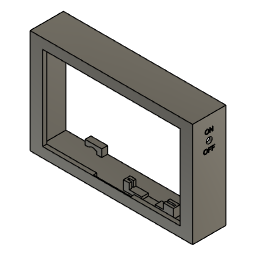
display (Autodesk Fusion 360 design; units mm, degrees)
Autodesk Fusion 360 part; units mm, degrees
note: some values were not read from the file. Set by a fixed rule: which face or edge a step refers to.
sketch "Outer" plane through (0, 0, 0) normal (0, 1, 0) x (1, 0, 0)
  line L0 (0, -125) -> (195, -125)
  line L1 (195, -125) -> (195, 0)
  line L2 (195, 0) -> (0, 0)
  line L3 (0, 0) -> (0, -125)
  line L4 (0, -62.5) -> (195, -62.5) construction
  line L5 (97.5, -125) -> (97.5, 0) construction
  dimension "d1" = 125
  dimension "d42" = 195
  constraint horizontal L0
  constraint vertical L1
  constraint horizontal L2
  constraint vertical L3
  constraint coincident L2.end L3.start
  constraint midpoint L3 L4.start
  constraint midpoint L1 L4.end
  constraint midpoint L0 L5.start
  constraint midpoint L2 L5.end
  measures "d1" distance of L0.start L2.end
  measures "d42" distance of L0.start L0.end
extrude "Extrude2" add sketch "Outer" along normal blind 40
shell "Shell1" thickness 3 removed faces 1 at (65, 40, 83.3333)
sketch "Screen Hole" plane through (0, 0, 0) normal (0, 1, 0) x (1, 0, 0)
  line L0 (15, -113) -> (180, -113)
  line L1 (180, -113) -> (180, -12)
  line L2 (180, -12) -> (15, -12)
  line L3 (15, -12) -> (15, -113)
  line L4 (0, -62.5) -> (195, -62.5)
  line L5 (0, 0) -> (0, -125)
  line L6 (3, -3) -> (3, -122)
  line L7 (192, -122) -> (192, -3)
  line L8 (97.5, -125) -> (97.5, 0)
  dimension "d10" = 165
  dimension "d11" = 101
  constraint horizontal L0
  constraint vertical L1
  constraint horizontal L2
  constraint vertical L3
  constraint symmetric L0 L2 L4
  constraint symmetric L1 L3 L8
  measures "d10" distance of L0.start L0.end
  measures "d11" distance of L0.start L2.end
extrude "Extrude3" cut sketch "Screen Hole" along normal blind 10
move_face "OffsetFaces1" offset 2 1 faces at (7, 3, 45.6667)
sketch "Cable Wedge" plane through (0, 5, 0) normal (0, 1, 0) x (-1, 0, 0)
  line L0 (-15, 12) -> (-180, 12)
  line L1 (-180, 12) -> (-180, 113)
  line L2 (-180, 113) -> (-15, 113)
  line L3 (-15, 113) -> (-15, 12)
  line L4 (-3, 3) -> (-3, 122)
  line L5 (-3, 122) -> (-192, 122)
  line L6 (-192, 122) -> (-192, 3)
  line L7 (-192, 3) -> (-3, 3)
  line L8 (-120, 12) -> (-75, 12)
  line L9 (-75, 12) -> (-75, 8)
  line L10 (-75, 8) -> (-120, 8)
  line L11 (-120, 8) -> (-120, 12)
  line L12 (-180, 113) -> (-180, 12)
  dimension "d43" = 60
  dimension "d44" = 45
  dimension "d45" = 4
  constraint horizontal L8
  constraint vertical L9
  constraint horizontal L10
  constraint vertical L11
  constraint coincident L0 L8.start
  measures "d43" distance of L11 L12
  measures "d44" distance of L9 L11
  measures "d45" distance of L8.start L10.end
extrude "Extrude6" cut sketch "Cable Wedge" against normal blind 4 contours L0 L8 L9 L10 L11
sketch "Screw Holes" plane through (0, 5, 0) normal (0, 1, 0) x (-1, 0, 0)
  line L0 (-120, 12) -> (-180, 12)
  line L1 (-180, 12) -> (-180, 113)
  line L2 (-180, 113) -> (-15, 113)
  line L3 (-15, 113) -> (-15, 12)
  line L4 (-3, 3) -> (-3, 122)
  line L5 (-3, 122) -> (-192, 122)
  line L6 (-192, 122) -> (-192, 3)
  line L7 (-192, 3) -> (-3, 3)
  circle A0 centre (-18.937, 8.19) radius 1.219
  circle A1 centre (-176.063, 8.19) radius 1.219
  circle A2 centre (-176.063, 116.81) radius 1.219
  circle A3 centre (-18.937, 116.81) radius 1.219
  line L8 (-120, 8) -> (-120, 12)
  line L9 (-15, 12) -> (-75, 12)
  line L10 (-75, 12) -> (-75, 8)
  line L11 (-75, 8) -> (-120, 8)
  dimension "d16" = 2.438
  dimension "d24" = 3.81
  dimension "d26" = 2.438
  dimension "d28" = 3.937
  dimension "d29" = 3.937
  dimension "d30" = 3.81
  dimension "d31" = 2.438
  dimension "d32" = 3.81
  dimension "d33" = 3.937
  dimension "d34" = 2.438
  dimension "d35" = 3.81
  dimension "d36" = 3.937
  measures "d16" diameter of A0
  measures "d24" distance of L0 A0.centre
  measures "d26" diameter of A1
  measures "d28" distance of L3 A0.centre
  measures "d29" distance of L1 A1.centre
  measures "d30" distance of L0 A1.centre
  measures "d31" diameter of A2
  measures "d32" distance of L2 A2.centre
  measures "d33" distance of L1 A2.centre
  measures "d34" diameter of A3
  measures "d35" distance of L2 A3.centre
  measures "d36" distance of L3 A3.centre
extrude "Extrude5" cut sketch "Screw Holes" against normal blind 4 contours A0 | A1 | A2 | A3
sketch "Switch Hole" plane through (195, 0, 0) normal (1, 0, 0) x (0, 1, 0)
  line L0 (0, 125) -> (0, 0)
  line L1 (0, 0) -> (40, 0)
  line L2 (40, 0) -> (40, 125)
  line L3 (40, 125) -> (0, 125)
  circle A0 centre (19.9992, 98.5) radius 3.5
  line L4 (5, 122) -> (40, 122)
  line L5 (20, 102) -> (20, 95) construction
  dimension "d49" = 7
  dimension "d56" = 20
  constraint coincident A0 L5.start
  constraint coincident A0 L5.end
  constraint parallel L2 L5
  constraint symmetric L0 L2 L5
  measures "d49" diameter of A0
  measures "d56" distance of A0 L4
extrude "Extrude7" cut sketch "Switch Hole" against normal blind 3 contours A0
sketch "Switch Text" plane through (195, 0, 0) normal (1, 0, 0) x (0, 1, 0)
  circle A0 centre (19.9992, 98.5) radius 3.5
  line L0 (0, 125) -> (0, 0)
  line L1 (0, 0) -> (40, 0)
  line L2 (40, 0) -> (40, 125)
  line L3 (40, 125) -> (0, 125)
  line L4 (15, 106) -> (25, 106) construction
  line L5 (25, 106) -> (25, 111) construction
  line L6 (25, 111) -> (15, 111) construction
  line L7 (15, 111) -> (15, 106) construction
  line L8 (20, 102) -> (20, 95)
  line L9 (13.25, 86) -> (26.75, 86) construction
  line L10 (26.75, 86) -> (26.75, 91) construction
  line L11 (26.75, 91) -> (13.25, 91) construction
  line L12 (13.25, 91) -> (13.25, 86) construction
  circle A1 centre (19.9992, 98.5) radius 3.5
  dimension "d57" = 5
  dimension "d58" = 5
  dimension "d59" = 10
  dimension "d60" = 5
  dimension "d61" = 5
  dimension "d62" = 13.5
  dimension "d64" = 4
  dimension "d65" = 4
  text T0 "ON" font "Arial" height 5 align left top in box 10 x 5 at (15, 106) x (1, 0) y (0, 1) spacing 1 kerned
  text T1 "OFF\n" font "Arial" height 5 align left top in box 13.5 x 5 at (13.25, 86) x (1, 0) y (0, 1) spacing 1 kerned
  constraint vertical L5
  constraint vertical L10
extrude "Extrude8" cut sketch "Switch Text" against normal blind 2 text T0 T1
sketch "Cable Holder" plane through (0, 40, 0) normal (0, 1, 0) x (-1, 0, 0)
  line L0 (-3, 3) -> (-192, 3)
  line L1 (-192, 3) -> (-192, 122)
  line L2 (-192, 122) -> (-3, 122)
  line L3 (-3, 122) -> (-3, 3)
  line L4 (0, 0) -> (0, 125)
  line L5 (0, 125) -> (-195, 125)
  line L6 (-195, 125) -> (-195, 0)
  line L7 (-195, 0) -> (0, 0)
  line L8 (-53, 3) -> (-53, 12)
  line L9 (-53, 12) -> (-33, 12)
  line L10 (-33, 12) -> (-33, 6)
  line L11 (-33, 6) -> (-37, 6)
  line L12 (-47, 6) -> (-47, 3)
  line L13 (-53, 3) -> (-47, 3)
  spline S0 degree 5 poles (-47, 6) (-46.8, 6.1517) (-46.4, 6.4418) (-45.8, 6.8373) (-45, 7.2838) (-44, 7.6981) (-43, 7.9558) (-42, 8.044) (-41, 7.9558) (-40, 7.6981) (-39, 7.2838) (-38.2, 6.8373) (-37.6, 6.4418) (-37.2, 6.1517) (-37, 6) knots 0 0 0 0 0 0 0.1 0.2 0.3 0.4 0.5 0.6 0.7 0.8 0.9 1 1 1 1 1 1
  point P0 (-42, 8)
  dimension "d69" = 3
  dimension "d70" = 9
  dimension "d71" = 5
  dimension "d72" = 4
  dimension "d73" = 6
  dimension "d74" = 10
  dimension "d75" = 30
  dimension "d76" = 5
  dimension "d96" = 3
  constraint coincident L0 L8.start
  constraint perpendicular L0 L8
  constraint perpendicular L8 L9
  constraint perpendicular L9 L10
  constraint perpendicular L10 L11
  constraint coincident L0 L12.end
  constraint perpendicular L0 L12
  measures "d69" distance of L0 L11
  measures "d70" distance of L8.start L8.end
  measures "d71" distance of L0 P0
  measures "d72" distance of L10.end L11.end
  measures "d73" distance of L8.start L12.end
  measures "d74" distance of L11.end L12
  measures "d75" distance of L3 L10
  measures "d76" horizontal distance of L12.start P0
  measures "d96" distance of L12.start L12.end
extrude "Extrude9" add sketch "Cable Holder" against normal blind 7 contours L0 L8 L9 L10 L11 L12 L13 S0
ref_plane "WorkPlane6" through (97.5, 20, 62.5) normal (0, 1, 0) x (1, 0, 0)
sketch "Pi Holder" plane through (97.5, 20, 62.5) normal (0, 1, 0) x (-1, 0, 0)
  line L0 (-50.5, -55.5) -> (-50.5, -48.5)
  line L1 (-50.5, -48.5) -> (-60.5, -48.5)
  line L2 (-60.5, -48.5) -> (-60.5, -59.5) construction
  line L3 (-4.5, -59.5) -> (-4.5, -48.5) construction
  line L4 (-4.5, -48.5) -> (-9.5, -48.5)
  line L5 (-9.5, -48.5) -> (-9.5, -55.5)
  line L6 (44.5, -59.5) -> (-94.5, -59.5)
  line L7 (-82.5, -50.5) -> (-82.5, 50.5)
  line L8 (-4.5, -59.5) -> (-60.5, -59.5)
  line L9 (-50.5, -55.5) -> (-40.5, -55.5)
  line L10 (-40.5, -55.5) -> (-40.5, -58.5)
  line L11 (-40.5, -58.5) -> (-24.5, -58.5)
  line L12 (-24.5, -58.5) -> (-24.5, -55.5)
  line L13 (-24.5, -55.5) -> (-9.5, -55.5)
  line L14 (-62.5, -48.5) -> (-60.5, -48.5)
  line L15 (-62.5, -59.5) -> (-62.5, -48.5)
  line L16 (-4.5, -48.5) -> (-2.5, -48.5)
  line L17 (-2.5, -48.5) -> (-2.5, -59.5)
  line L18 (-2.5, -59.5) -> (-4.5, -59.5)
  line L19 (-62.5, -59.5) -> (-60.5, -59.5)
  dimension "d82" = 5
  dimension "d84" = 56
  dimension "d97" = 10
  dimension "d98" = 7
  dimension "d99" = 7
  dimension "d100" = 3
  dimension "d101" = 3
  dimension "d104" = 20
  dimension "d105" = 20
  dimension "d106" = 1
  dimension "d107" = 2
  dimension "d108" = 2
  dimension "d109" = 20
  constraint vertical L0
  constraint horizontal L1
  constraint vertical L2
  constraint vertical L3
  constraint horizontal L4
  constraint vertical L5
  constraint horizontal L8
  constraint collinear L6 L8
  constraint perpendicular L0 L9
  constraint perpendicular L1 L10
  constraint perpendicular L10 L11
  constraint perpendicular L11 L12
  constraint perpendicular L5 L13
  constraint horizontal L14
  constraint vertical L15
  constraint coincident L1.end L2.start
  constraint horizontal L16
  constraint vertical L17
  constraint horizontal L18
  constraint coincident L6 L15.start
  measures "d82" distance of L3.end L4.end
  measures "d84" distance of L2 L3
  measures "d97" distance of L0.end L1.end
  measures "d98" distance of L0.start L0.end
  measures "d99" distance of L5.end L4.end
  measures "d100" distance of L9.end L10.end
  measures "d101" distance of L11.end L12.end
  measures "d104" distance of L2 L10
  measures "d105" distance of L3 L12
  measures "d106" distance of L8 L11
  measures "d107" distance of L14.start L1.end
  measures "d108" distance of L3.end L16.end
  measures "d109" distance of L7 L15
extrude "Extrude10" add sketch "Pi Holder" against normal blind 8
sketch "Pi Holder Holes" plane through (97.5, 20, 62.5) normal (0, 1, 0) x (1, 0, 0)
  line L0 (9.5, 48.5) -> (4.5, 48.5)
  line L1 (4.5, 48.5) -> (4.5, 55.5)
  line L2 (4.5, 55.5) -> (9.5, 55.5)
  line L3 (9.5, 55.5) -> (9.5, 48.5)
  line L4 (60.5, 48.5) -> (50.5, 48.5)
  line L5 (50.5, 48.5) -> (50.5, 55.5)
  line L6 (50.5, 55.5) -> (60.5, 55.5)
  line L7 (60.5, 55.5) -> (60.5, 48.5)
  point P0 (9.5, 55.5)
  point P1 (4.5, 48.5)
  point P2 (60.5, 48.5)
  point P3 (50.5, 55.5)
  constraint horizontal L0
  constraint vertical L1
  constraint horizontal L2
  constraint vertical L3
  constraint coincident P0 L2.end
  constraint coincident P1 L0.end
  constraint horizontal L4
  constraint vertical L5
  constraint horizontal L6
  constraint vertical L7
  constraint coincident P2 L4.start
  constraint coincident P3 L5.end
extrude "Extrude11" cut sketch "Pi Holder Holes" against normal blind 2 from surface at -3
